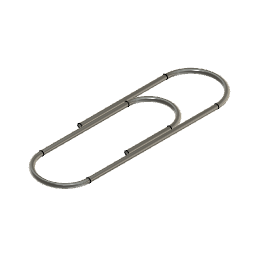
gyakorlati 2 gemkapocs (Autodesk Fusion 360 design; units mm, degrees)
Autodesk Fusion 360 part; units mm, degrees
sketch "Sketch1" plane through (0, 0, 0) normal (0, 0, 1) x (1, 0, 0)
  line L0 (0, 0) -> (0, 50)
  line L1 (50, 50) -> (50, 0)
  arc A0 (50, 50) -> (0, 50) centre (25, 50) ccw
  line L2 (-5, 100) -> (-5, 0)
  line L3 (55, 100) -> (55, 0)
  line L4 (55, 0) -> (55, -50)
  line L5 (0, 0) -> (0, -50)
  arc A1 (55, 100) -> (-5, 100) centre (25, 100) ccw
  arc A2 (0, -50) -> (55, -50) centre (27.5, -50) ccw
  constraint coincident L0.start L5.start
  constraint vertical L0
  constraint tangent L1 A0
  constraint tangent L0 A0
  constraint parallel L0 L2
  constraint vertical L3
  constraint parallel L3 L4
  constraint parallel L0 L5
  constraint tangent L3 A1
  constraint tangent L2 A1
  constraint tangent L5 A2
pipe "Pipe1" add diameter 5 path "Sketch1" along L1 A0 L0 L5 A2 L4 L3 A1 L2
